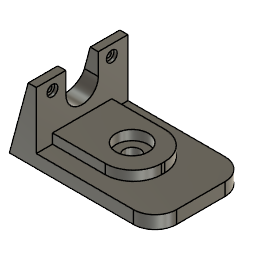
ex2 (Autodesk Fusion 360 design; units mm, degrees)
part number: 2026-04-20-19-02-57-717
Autodesk Fusion 360 part; units mm, degrees
sketch "Baza" plane through (0, 0, 0) normal (0, 0, 1) x (1, 0, 0)
  line L0 (0, 0) -> (0, 85)
  line L1 (0, 85) -> (135, 85)
  line L2 (135, 85) -> (135, 0)
  line L3 (135, 0) -> (0, 0)
  line L4 (0, 0) -> (25, 0) construction
  line L5 (25, 0) -> (25, 85)
  line L6 (25, 85) -> (25, 70) construction
  line L7 (25, 0) -> (25, 15) construction
  line L8 (69.701, 85) -> (69.701, 0) construction
  line L9 (135, 85) -> (69.701, 44.195) construction
  circle A0 centre (69.701, 44.195) radius 7.5
  circle A1 centre (69.701, 44.195) radius 15
  line L10 (25, 70) -> (100, 70)
  line L11 (100, 70) -> (100, 15)
  line L12 (100, 15) -> (25, 15)
  line L13 (25, 15) -> (25, 70)
  dimension "d1" = 85
  dimension "d2" = 135
  dimension "d3" = 25
  dimension "d4" = 15
  dimension "d5" = 15
  dimension "d6" = 77
  dimension "d7" = 15
  dimension "d8" = 30
  dimension "d9" = 55
  dimension "d10" = 44.701
  dimension "d11" = 35
  constraint coincident L0.start L3.end
  constraint vertical L0
  constraint perpendicular L0 L1
  constraint perpendicular L1 L2
  constraint perpendicular L0 L3
  constraint perpendicular L0 L4
  constraint coincident L1 L5.end
  constraint perpendicular L1 L5
  constraint perpendicular L1 L6
  constraint perpendicular L4 L7
  constraint coincident L1 L8.start
  constraint coincident L3 L8.end
  constraint perpendicular L3 L8
  constraint coincident L8 L9.end
  constraint coincident L9.end A0.centre
  constraint concentric A0 A1
  constraint horizontal L10
  constraint vertical L11
  constraint horizontal L12
  constraint vertical L13
  measures "d1" distance of L0.start L0.end
  measures "d2" distance of L0.end L1.end
  measures "d3" distance of L0.start L4.end
  measures "d4" distance of L5.end L6.end
  measures "d5" distance of L4.end L7.end
  measures "d6" distance of L1.end L9.end
  measures "d7" diameter of A0
  measures "d8" diameter of A1
  measures "d9" distance of L10 L12
  measures "d10" distance of L5 L9.end
  measures "d11" distance of L2 L11
extrude "Extrude1" add sketch "Baza" along normal blind 12 contours L0 L1 L3 L5 L13 | L1 L2 L3 L5 L10 L11 L12 | L5 L10 L11 L12 L13 | A0 | A1 makes body 1
extrude "Extrude2" add sketch "Baza" along normal blind 21 separate body contours L5 L10 L11 L12 L13 makes body 2
combine "Combine1" operation add target body 2 tool bodies 1
extrude "Extrude3" cut sketch "Baza" along normal blind 50 contours A0 bodies 2
fillet "Fillet1" radius 26 2 edges at (100, 15, 16.5) (100, 70, 16.5) on bodies 2
fillet "Fillet2" radius 20 2 edges at (135, 0, 6) (135, 85, 6) on bodies 2
sketch "Margine" plane through (0, 0, 0) normal (0, -1, 0) x (1, 0, 0)
  line L0 (115, 0) -> (115, 12)
  line L1 (115, 12) -> (0, 12)
  line L2 (0, 12) -> (0, 0)
  line L3 (0, 0) -> (115, 0)
  line L4 (0, 0) -> (25, 0) construction
  line L5 (25, 0) -> (25, 65)
  line L6 (0, 0) -> (17.3848, 64.881)
  line L7 (0, 0) -> (67.1698, 0) construction
  line L8 (17.3848, 64.881) -> (25, 65)
  line L9 (3.2154, 12) -> (25, 12)
  line L10 (3.2154, 12) -> (0, 12)
  line L11 (0, 0) -> (0, 12)
  dimension "d22" = 25
  dimension "d23" = 65
  dimension "d24" = 75
  constraint coincident L2.end L3.start
  constraint perpendicular L2 L4
  constraint perpendicular L4 L5
  constraint horizontal L7
  constraint coincident L6 L9.start
  constraint coincident L1 L9.start
  constraint coincident L5 L9.end
  constraint coincident L1 L9.end
  constraint coincident L1.end L2.start
  measures "d22" distance of L2.end L4.end
  measures "d23" distance of L4.end L5.end
  measures "d24" angle of L6 L7
extrude "Extrude4" add sketch "Margine" against normal blind 85 contours L1 L5 L6 L8 L9 bodies 2
extrude "Extrude5" cut sketch "Margine" against normal blind 85 contours L1 L2 L6 L10 L11 bodies 2
sketch "Fata" plane through (25, 0, 0) normal (1, 0, 0) x (0, 1, 0)
  line L0 (70, 21) -> (70, 12)
  line L1 (70, 12) -> (85, 12)
  line L2 (85, 12) -> (85, 65)
  line L3 (85, 65) -> (0, 65)
  line L4 (0, 65) -> (0, 12)
  line L5 (0, 12) -> (15, 12)
  line L6 (15, 12) -> (15, 21)
  line L7 (15, 21) -> (70, 21)
  line L8 (0, 65) -> (15, 65) construction
  line L9 (85, 65) -> (70, 65) construction
  line L10 (15, 65) -> (15, 55) construction
  line L11 (70, 65) -> (70, 55) construction
  circle A0 centre (15, 55) radius 2.5
  circle A1 centre (70, 55) radius 2.5
  circle A2 centre (15, 55) radius 5
  circle A3 centre (70, 55) radius 5
  line L12 (0, 65) -> (0, 45) construction
  line L13 (0, 45) -> (85, 45) construction
  line L14 (27.5, 45) -> (27.5, 65)
  line L15 (57.5, 45) -> (57.5, 65)
  arc A4 (27.5, 45) -> (57.5, 45) centre (42.5, 45) ccw
  dimension "d29" = 15
  dimension "d30" = 15
  dimension "d31" = 10
  dimension "d32" = 10
  dimension "d33" = 5
  dimension "d34" = 5
  dimension "d35" = 10
  dimension "d36" = 10
  dimension "d37" = 20
  dimension "d40" = 30
  constraint coincident L3.end L4.start
  constraint coincident L3 L8.end
  constraint coincident L2.end L3.start
  constraint perpendicular L2 L9
  constraint perpendicular L3 L10
  constraint perpendicular L9 L11
  constraint coincident L10.end A0.centre
  constraint coincident L11.end A1.centre
  constraint concentric A0 A2
  constraint concentric A1 A3
  constraint perpendicular L8 L12
  constraint coincident L2 L13.end
  constraint perpendicular L2 L13
  constraint midpoint L13 A4.centre
  constraint coincident L13 L14.start
  constraint coincident L3 L14.end
  constraint tangent L14 A4
  constraint coincident L13 L15.start
  constraint coincident L3 L15.end
  constraint tangent L15 A4
  measures "d29" distance of L3.end L8.end
  measures "d30" distance of L2.end L9.end
  measures "d31" distance of L8.end L10.end
  measures "d32" distance of L9.end L11.end
  measures "d33" diameter of A0
  measures "d34" diameter of A1
  measures "d35" diameter of A2
  measures "d36" diameter of A3
  measures "d37" distance of L3.end L12.end
  measures "d40" diameter of A4
extrude "Extrude6" cut sketch "Fata" against normal blind 20 contours L3 L14 L15 A4 bodies 2
extrude "Extrude7" cut sketch "Fata" against normal blind 15 contours A0 | A1 bodies 2
extrude "Extrude8" cut sketch "Fata" against normal blind 3 contours A2 | A3 bodies 2
named bodies: "Baza", "Piesa"
